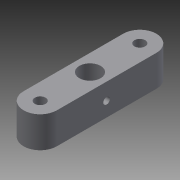
# Autodesk Inventor part: throwing_motor_support
Saved by Autodesk Inventor 2015 (Build 190159000, 159)
## iProperties
Created: 2017-12-15
Part Number: throwing_motor_support
Material: Generic
Document SubType Name: Modeling
Designer: Anshul
Density: 1 g/cm^3
Appearance: Default
Author: Anshul
Autodesk Inventor part; units mm, degrees
ref_plane "YZ Plane" through (0, 0, 0) normal (1, 0, 0) x (0, 1, 0)
ref_plane "XZ Plane" through (0, 0, 0) normal (0, 1, 0) x (-1, 0, 0)
ref_plane "XY Plane" through (0, 0, 0) normal (0, 0, 1) x (1, 0, 0)
sketch "Sketch1" plane through (0, 0, 0) normal (0, 1, 0) x (-1, 0, 0)
  circle A0 centre (0, 0) radius 3.15
  circle A1 centre (0, 0) radius 5.15
  line L0 (0, 0) -> (0, -24)
  line L1 (0, 0) -> (0, 24)
  circle A2 centre (0, 24) radius 2.6
  circle A3 centre (0, -24) radius 2.6
  line L2 (8, 24) -> (8, -24)
  line L3 (-8, 24) -> (-8, -24)
  circle A4 centre (0, 24) radius 4
  circle A5 centre (0, -24) radius 4
  line L4 (4, 17.0718) -> (4, 6.9282)
  line L5 (-4, 17.0718) -> (-4, 6.9282)
  line L6 (4, -17.0718) -> (4, -6.9282)
  line L7 (-4, -17.0718) -> (-4, -6.9282)
  arc A6 (-8, -24) -> (8, -24) centre (0, -24) ccw
  arc A7 (4, -17.0718) -> (-4, -17.0718) centre (0, -24) ccw
  arc A8 (8, 24) -> (-8, 24) centre (0, 24) ccw
  arc A9 (-4, 17.0718) -> (4, 17.0718) centre (0, 24) ccw
  arc A10 (4, 6.9282) -> (-4, 6.9282) centre (0, 0) ccw
  arc A11 (-4, -6.9282) -> (4, -6.9282) centre (0, 0) ccw
  dimension "d0" = 6.3
  dimension "d5" = 10.3
  dimension "d15" = 24
  dimension "d16" = 24
  dimension "d17" = 5.2
  dimension "d18" = 5.2
  dimension "d22" = 8
  dimension "d23" = 8
  constraints: 16 end point, 12 centre point, 12 point on circle, 8 coincident, 4 tangent, 3 point on line, 2 vertical, 1 parallel
  measures "d0" diameter of A0
  measures "d5" diameter of A1
  measures "d15" distance of L0.start L0.end
  measures "d16" distance of L0.start L1.end
  measures "d17" diameter of A2
  measures "d18" diameter of A3
  measures "d22" diameter of A4
  measures "d23" diameter of A5
extrude "Extrusion3" add sketch "Sketch1" along normal blind 15 contours A5 | A11 L6 A7 L0 | L0 A7 L7 A11 | A4 | A10 L5 A9 L1 | L1 A9 L4 A10 | L2 A6 L3 A8
sketch "Sketch3" plane through (8, 0, 24) normal (1, 0, 0) x (0, 0, -1)
  line L0 (24, 0) -> (24, 7)
  circle A0 centre (24, 7) radius 1.6
  dimension "d26" = 7
  dimension "d27" = 3.2
  constraints: 2 end point, 1 centre point, 1 coincident, 1 vertical
  measures "d26" distance of L0.start L0.end
  measures "d27" diameter of A0
extrude "Extrusion4" cut sketch "Sketch3" against normal blind 30
body "Solid2"
